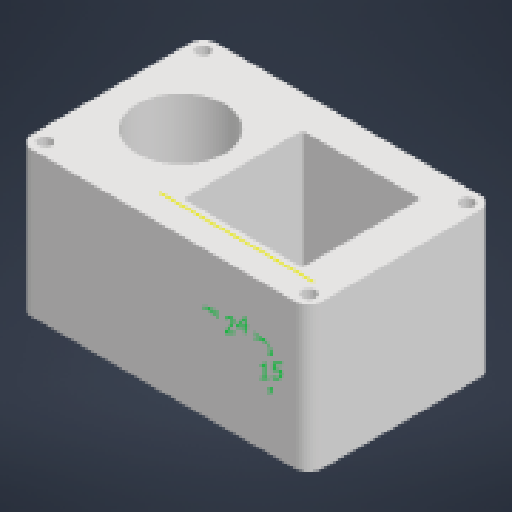
# Autodesk Inventor part: project_base
Saved by Autodesk Inventor 2024.2 (Build 282272000, 272)
## iProperties
Created: 2024-03-07
Part Number: project_base
Material: Generic
Document SubType Name: Modeling
Designer: seifs
Density: 1 g/cm^3
Appearance: Default
Author: seifs
Autodesk Inventor part; units mm, degrees
ref_plane "YZ Plane" through (0, 0, 0) normal (1, 0, 0) x (0, 1, 0)
ref_plane "XZ Plane" through (0, 0, 0) normal (0, 1, 0) x (-1, 0, 0)
ref_plane "XY Plane" through (0, 0, 0) normal (0, 0, 1) x (1, 0, 0)
sketch "Sketch1" plane through (0, 0, 0) normal (0, 1, 0) x (-1, 0, 0)
  line L0 (55, -35) -> (-55, -35)
  line L1 (-55, -35) -> (-55, 35)
  line L2 (-55, 35) -> (55, 35)
  line L3 (55, 35) -> (55, -35)
  line L4 (55, -35) -> (-55, 35) construction
  line L5 (-55, -35) -> (55, 35) construction
  point P0 (0, 0)
  dimension "d143" = 110
  dimension "d144" = 70
  constraints: 12 end point, 2 midpoint, 2 parallel, 1 horizontal, 1 perpendicular
  measures "d143" distance of L1.end L2.end
  measures "d144" distance of L0.end L1.end
extrude "Extrusion1" add sketch "Sketch1" along normal blind 10
sketch "Sketch2" plane through (0, 10, 0) normal (0, 1, 0) x (1, 0, 0)
  line L0 (50, 30) -> (-50, -30) construction
  line L1 (50, 0) -> (17.5, 0) construction
  line L2 (-3, 22.5) -> (38, 22.5)
  line L3 (40, 20.5) -> (40, -20.5)
  line L4 (38, -22.5) -> (-3, -22.5)
  line L5 (-5, -20.5) -> (-5, 20.5)
  line L6 (-5, 22.5) -> (40, -22.5) construction
  line L7 (40, 22.5) -> (-5, -22.5) construction
  arc A0 (-3, 22.5) -> (-5, 20.5) centre (-3, 20.5) ccw
  arc A1 (-5, -20.5) -> (-3, -22.5) centre (-3, -20.5) ccw
  arc A2 (38, -22.5) -> (40, -20.5) centre (38, -20.5) ccw
  arc A3 (40, 20.5) -> (38, 22.5) centre (38, 20.5) ccw
  line L8 (-5.5, 25) -> (40.5, 25)
  line L9 (42.5, 23) -> (42.5, -23)
  line L10 (40.5, -25) -> (-5.5, -25)
  line L11 (-7.5, -23) -> (-7.5, 23)
  line L12 (-7.5, 25) -> (42.5, -25) construction
  line L13 (42.5, 25) -> (-7.5, -25) construction
  arc A4 (-5.5, 25) -> (-7.5, 23) centre (-5.5, 23) ccw
  arc A5 (42.5, 23) -> (40.5, 25) centre (40.5, 23) ccw
  arc A6 (40.5, -25) -> (42.5, -23) centre (40.5, -23) ccw
  arc A7 (-7.5, -23) -> (-5.5, -25) centre (-5.5, -23) ccw
  line L14 (-5, 0) -> (-28.5, 0) construction
  circle A8 centre (-28.5, 0) radius 16.5
  circle A9 centre (-28.5, 0) radius 18.5
  point P0 (0, 0)
  dimension "d122" = 32.5
  dimension "d123" = 45
  dimension "d124" = 45
  dimension "d125" = 2
  dimension "d126" = 2
  dimension "d127" = 2
  dimension "d128" = 2
  dimension "d129" = 50
  dimension "d130" = 50
  dimension "d131" = 2
  dimension "d132" = 23.5
  dimension "d133" = 33
  dimension "d134" = 37
  constraints: 30 end point, 16 point on circle, 16 point on line, 16 tangent, 10 centre point, 6 midpoint, 4 horizontal, 4 parallel, 3 equal radius, 2 coincident, 2 perpendicular
  measures "d122" distance of L1.start L1.end
  measures "d123" distance of L6.end L7.end
  measures "d124" distance of L7.start L6.end
  measures "d125" radius of A0
  measures "d126" radius of A1
  measures "d127" radius of A2
  measures "d128" radius of A3
  measures "d129" distance of L12.end L13.end
  measures "d130" distance of L13.start L12.end
  measures "d131" radius of A4
  measures "d132" distance of L14.start L14.end
  measures "d133" diameter of A8
  measures "d134" diameter of A9
extrude "Extrusion2" add sketch "Sketch2" along normal blind 45
sketch "Sketch10" plane through (0, 55, 0) normal (0, 1, 0) x (1, 0, 0)
  line L0 (0, 0) -> (-5, 0) construction
  line L1 (-4, 22.5) -> (39, 22.5)
  line L2 (40, 21.5) -> (40, -21.5)
  line L3 (39, -22.5) -> (-4, -22.5)
  line L4 (-5, -21.5) -> (-5, 21.5)
  line L5 (-5, 22.5) -> (40, -22.5) construction
  line L6 (40, 22.5) -> (-5, -22.5) construction
  arc A0 (-4, 22.5) -> (-5, 21.5) centre (-4, 21.5) ccw
  arc A1 (-5, -21.5) -> (-4, -22.5) centre (-4, -21.5) ccw
  arc A2 (39, -22.5) -> (40, -21.5) centre (39, -21.5) ccw
  arc A3 (40, 21.5) -> (39, 22.5) centre (39, 21.5) ccw
  point P0 (17.5, 0)
  dimension "d71" = 5
  dimension "d73" = 45
  dimension "d74" = 1
  constraints: 14 end point, 8 point on circle, 8 point on line, 8 tangent, 4 centre point, 3 equal radius, 2 horizontal, 2 midpoint, 2 parallel, 1 perpendicular
  measures "d71" distance of L0.start L0.end
  measures "d73" distance of L6.start L5.end
  measures "d74" radius of A0
extrude "Extrusion8" cut sketch "Sketch10" against normal blind 45
sketch "Sketch11" plane through (0, 55, 0) normal (0, 1, 0) x (1, 0, 0)
  line L0 (-5, -21.5) -> (-5, 21.5) projected
  line L1 (-5, 0) -> (-5, 15.5)
  line L2 (-50, 30) -> (-50, -30) projected
  circle A0 centre (-10, 15.5) radius 1.5
  line L3 (-4, 22.5) -> (39, 22.5) projected
  circle A1 centre (-10, -15.5) radius 1.5
  circle A2 centre (45, 15.5) radius 1.5
  circle A3 centre (45, -15.5) radius 1.5
  arc A4 (-5.5, 25) -> (-7.5, 23) centre (-5.5, 23) ccw projected
  line L4 (-5.5, 25) -> (-11.5, 25)
  circle A5 centre (-28.5, 0) radius 18.5 projected
  arc A6 (-13.5, -10.8282) -> (-13.5, 10.8282) centre (-28.5, 0) ccw
  line L5 (-13.5, 23) -> (-13.5, 10.8282)
  line L6 (-13.5, -10.8282) -> (-13.5, -23)
  line L7 (40.5, -25) -> (-5.5, -25) projected
  line L8 (-11.5, -25) -> (-5.5, -25)
  arc A7 (-11.5, 25) -> (-13.5, 23) centre (-11.5, 23) ccw
  arc A8 (-13.5, -23) -> (-11.5, -25) centre (-11.5, -23) ccw
  arc A9 (42.5, 23) -> (40.5, 25) centre (40.5, 23) ccw projected
  line L9 (40.5, 25) -> (46.5, 25)
  line L10 (48.5, 23) -> (48.5, -23)
  line L11 (46.5, -25) -> (40.5, -25)
  arc A10 (48.5, 23) -> (46.5, 25) centre (46.5, 23) ccw
  arc A11 (46.5, -25) -> (48.5, -23) centre (46.5, -23) ccw
  line L12 (-5.5, 25) -> (-5.5, -25)
  line L13 (40.5, 25) -> (-5.5, 25) projected
  line L14 (40.5, 25) -> (40.5, -25)
  line L15 (42.5, -23) -> (42.5, 23) projected
  point P0 (0, 0)
  point P1 (-50, 24.2086)
  point P2 (-50, -24.2086)
  point P3 (-50, 28)
  point P4 (-50, -28)
  point P5 (-13.5, 25)
  point P6 (48.5, 25)
  dimension "d79" = 3
  dimension "d135" = 8
  dimension "d136" = 2
  dimension "d137" = 8
  dimension "d138" = 2
  constraints: 20 end point, 12 point on circle, 10 tangent, 9 centre point, 5 point on line, 3 horizontal, 3 vertical, 2 equal radius, 2 perpendicular, 1 midpoint, 1 parallel
  measures "d79" diameter of A0
  measures "d135" distance of L4.start point (-13.5, 25)
  measures "d136" radius of A7
  measures "d137" distance of L9.start point (48.5, 25)
  measures "d138" radius of A10
extrude "Extrusion9" add sketch "Sketch11" against normal blind 5 contours L12 L8 A8 L6 A5 L5 A7 L4 | L9 A10 L10 A11 L11 L14
fillet "Fillet5" radius 5 4 edges at (-55, 5, 35) (55, 5, 35) (55, 5, -35) (-55, 5, -35)
sketch "Sketch19" plane through (0, 10, 0) normal (0, 1, 0) x (1, 0, 0)
  arc A0 (-55, -30) -> (-50, -35) centre (-50, -30) ccw projected
  circle A1 centre (-50, -30) radius 2.5
  arc A2 (-50, 35) -> (-55, 30) centre (-50, 30) ccw projected
  circle A3 centre (-50, 30) radius 2.5
  arc A4 (55, 30) -> (50, 35) centre (50, 30) ccw projected
  circle A5 centre (50, 30) radius 2.5
  arc A6 (50, -35) -> (55, -30) centre (50, -30) ccw projected
  circle A7 centre (50, -30) radius 2.5
  point P0 (0, 0)
  dimension "d146" = 5
  dimension "d147" = 5
  dimension "d148" = 5
  dimension "d149" = 5
  constraints: 4 centre point, 4 coincident
  measures "d146" diameter of A1
  measures "d147" diameter of A3
  measures "d148" diameter of A5
  measures "d149" diameter of A7
extrude "Extrusion13" cut sketch "Sketch19" against normal blind 10
sketch "Sketch20" plane through (-5.5, 10, 25) normal (0, 0, 1) x (1, 0, 0)
  line L0 (46, 0) -> (0, 0) projected
  line L1 (46, 0) -> (46, 40) projected
  line L2 (52, 40) -> (46, 40) projected
  line L3 (52, 45) -> (52, 40) projected
  line L4 (-6, 45) -> (52, 45) projected
  line L5 (-6, 45) -> (-6, 40) projected
  line L6 (0, 40) -> (-6, 40) projected
  line L7 (0, 0) -> (0, 40) projected
  line L8 (46, 0) -> (0, 0) projected
  line L9 (11, 0) -> (35, 0)
  line L10 (35, 0) -> (35, 15)
  line L11 (35, 15) -> (11, 15)
  line L12 (11, 15) -> (11, 0)
  point P0 (5.5, -10)
  dimension "d152" = 24
  dimension "d153" = 15
  constraints: 8 end point, 2 parallel, 1 horizontal, 1 perpendicular, 1 point on line
  measures "d152" distance of L11.end L10.end
  measures "d153" distance of L10.end L9.end
sketch "Sketch21" plane through (0, 10, 0) normal (0, 1, 0) x (1, 0, 0)
  circle A0 centre (50, -30) radius 2.5 projected
  circle A1 centre (-50, -30) radius 2.5 projected
  circle A2 centre (50, 30) radius 2.5 projected
  circle A3 centre (-50, 30) radius 2.5 projected
  arc A4 (-7.5, -23) -> (-5.5, -25) centre (-5.5, -23) ccw projected
  line L0 (-7.5, -23) -> (-7.5, 23) projected
  arc A5 (-5.5, 25) -> (-7.5, 23) centre (-5.5, 23) ccw projected
  line L1 (-5.5, 25) -> (40.5, 25) projected
  arc A6 (42.5, 23) -> (40.5, 25) centre (40.5, 23) ccw projected
  line L2 (42.5, 23) -> (42.5, -23) projected
  arc A7 (40.5, -25) -> (42.5, -23) centre (40.5, -23) ccw projected
  line L3 (40.5, -25) -> (-5.5, -25) projected
  circle A8 centre (-28.5, 0) radius 18.5 projected
  arc A9 (-50, 35) -> (-55, 30) centre (-50, 30) ccw projected
  line L4 (-55, 30) -> (-55, -30) projected
  arc A10 (-55, -30) -> (-50, -35) centre (-50, -30) ccw projected
  line L5 (-50, -35) -> (50, -35) projected
  arc A11 (50, -35) -> (55, -30) centre (50, -30) ccw projected
  line L6 (55, -30) -> (55, 30) projected
  arc A12 (55, 30) -> (50, 35) centre (50, 30) ccw projected
  line L7 (50, 35) -> (-50, 35) projected
  point P0 (0, 0)
extrude "Extrusion15" add sketch "Sketch21" along normal blind 40
extrude "Extrusion16" cut sketch "Sketch20" along normal blind 40 and the other way blind 5 contours L0 L12 L11 L10
sketch "Sketch22" plane through (0, 50, 0) normal (0, 1, 0) x (1, 0, 0)
  circle A0 centre (-50, -30) radius 2.5 projected
  line L0 (-55, 30) -> (-55, -30) projected
  line L1 (-55, -25) -> (-47, -25)
  line L2 (-55, -25) -> (-47, -25) construction
  line L3 (-45, -27) -> (-45, -35)
  line L4 (-50, -35) -> (50, -35) projected
  arc A1 (-45, -27) -> (-47, -25) centre (-47, -27) ccw
  line L5 (55, -25) -> (47, -25)
  line L6 (45, -27) -> (45, -35)
  arc A2 (47, -25) -> (45, -27) centre (47, -27) ccw
  line L7 (-55, 0) -> (0, 0) construction
  line L8 (-55, 25) -> (-47, 25)
  line L9 (-45, 27) -> (-45, 35)
  arc A3 (-47, 25) -> (-45, 27) centre (-47, 27) ccw
  line L10 (45, 27) -> (45, 35)
  line L11 (55, 25) -> (47, 25)
  arc A4 (45, 27) -> (47, 25) centre (47, 27) ccw
  arc A5 (-55, -30) -> (-50, -35) centre (-50, -30) ccw projected
  line L12 (-55, 30) -> (-55, -30) projected
  arc A6 (-50, 35) -> (-55, 30) centre (-50, 30) ccw projected
  line L13 (50, 35) -> (-50, 35) projected
  arc A7 (55, 30) -> (50, 35) centre (50, 30) ccw projected
  line L14 (55, -30) -> (55, 30) projected
  arc A8 (50, -35) -> (55, -30) centre (50, -30) ccw projected
  point P0 (-45, -25)
  dimension "d164" = 10
  dimension "d165" = 0
  dimension "d166" = 2
  constraints: 20 end point, 10 symmetric about line, 8 point on circle, 4 centre point, 4 point on line, 2 horizontal, 2 perpendicular, 2 tangent, 1 collinear, 1 midpoint, 2 other
  measures "d164" distance of L1.start point (-45, -25)
  measures "d165" distance between parallel lines of L1 L2
  measures "d166" radius of A1
extrude "Extrusion17" cut sketch "Sketch22" against normal blind 35 contours A6 L13 L9 A3 L8 L0 | L1 A1 L3 L4 A5 L0 | L13 A7 L14 L11 A4 L10 | L6 A2 L5 L14 A8 L4
fillet "Fillet7" radius 2 8 edges at (-55, 32.5, 25) (-45, 32.5, 35) (45, 32.5, 35) (55, 32.5, 25) (55, 32.5, -25) (45, 32.5, -35) (-45, 32.5, -35) (-55, 32.5, -25)
sketch "Sketch23" plane through (0, 50, 0) normal (0, 1, 0) x (1, 0, 0)
  arc A0 (-53, 25) -> (-55, 23) centre (-53, 23) ccw projected
  line L0 (-55, 23) -> (-55, -23) projected
  arc A1 (-55, -23) -> (-53, -25) centre (-53, -23) ccw projected
  line L1 (-53, -25) -> (-47, -25) projected
  arc A2 (-45, -27) -> (-47, -25) centre (-47, -27) ccw projected
  line L2 (-45, -27) -> (-45, -33) projected
  arc A3 (-45, -33) -> (-43, -35) centre (-43, -33) ccw projected
  line L3 (-43, -35) -> (43, -35) projected
  arc A4 (43, -35) -> (45, -33) centre (43, -33) ccw projected
  line L4 (45, -33) -> (45, -27) projected
  arc A5 (47, -25) -> (45, -27) centre (47, -27) ccw projected
  line L5 (47, -25) -> (53, -25) projected
  arc A6 (53, -25) -> (55, -23) centre (53, -23) ccw projected
  line L6 (55, -23) -> (55, 23) projected
  arc A7 (55, 23) -> (53, 25) centre (53, 23) ccw projected
  line L7 (53, 25) -> (47, 25) projected
  arc A8 (45, 27) -> (47, 25) centre (47, 27) ccw projected
  line L8 (45, 27) -> (45, 33) projected
  arc A9 (45, 33) -> (43, 35) centre (43, 33) ccw projected
  line L9 (43, 35) -> (-43, 35) projected
  arc A10 (-43, 35) -> (-45, 33) centre (-43, 33) ccw projected
  line L10 (-45, 33) -> (-45, 27) projected
  arc A11 (-47, 25) -> (-45, 27) centre (-47, 27) ccw projected
  line L11 (-47, 25) -> (-53, 25) projected
  line L12 (46.5, -25) -> (-11.5, -25) projected
  arc A12 (-13.5, -23) -> (-11.5, -25) centre (-11.5, -23) ccw projected
  line L13 (-13.5, -23) -> (-13.5, -10.8282) projected
  arc A13 (-13.5, 10.8282) -> (-13.5, -10.8282) centre (-28.5, 0) ccw projected
  line L14 (-13.5, 10.8282) -> (-13.5, 23) projected
  arc A14 (-11.5, 25) -> (-13.5, 23) centre (-11.5, 23) ccw projected
  line L15 (-11.5, 25) -> (46.5, 25) projected
  arc A15 (48.5, 23) -> (46.5, 25) centre (46.5, 23) ccw projected
  line L16 (48.5, 23) -> (48.5, -23) projected
  arc A16 (46.5, -25) -> (48.5, -23) centre (46.5, -23) ccw projected
  point P0 (0, 0)
extrude "Extrusion18" add sketch "Sketch23" along normal blind 5
body "Solid1"
